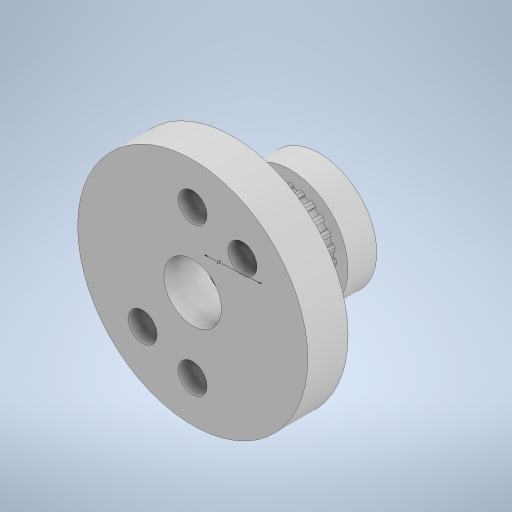
# Autodesk Inventor part: dondurgec
Saved by Autodesk Inventor 2023.2 (Build 272271000, 271)
## iProperties
Created: 2023-03-22
Part Number: dondurgec
Material: Generic
Document SubType Name: Modeling
Designer: sarp1
Density: 1 g/cm^3
Appearance: Default
Author: sarp1
Autodesk Inventor part; units mm, degrees
ref_plane "YZ Plane" through (0, 0, 0) normal (1, 0, 0) x (0, 1, 0)
ref_plane "XZ Plane" through (0, 0, 0) normal (0, 1, 0) x (-1, 0, 0)
ref_plane "XY Plane" through (0, 0, 0) normal (0, 0, 1) x (1, 0, 0)
sketch "Sketch1" plane through (0, 0, 0) normal (0, 0, 1) x (1, 0, 0)
  circle A0 centre (0, 0) radius 20
  circle A1 centre (0, 0) radius 5
  dimension "d0" = 40
  dimension "d1" = 10
  constraints: 2 centre point, 2 coincident
  measures "d0" diameter of A0
  measures "d1" diameter of A1
extrude "Extrusion1" add sketch "Sketch1" along normal blind 5 and the other way blind 2
sketch "Sketch2" plane through (0, 0, 5) normal (0, 0, 1) x (1, 0, 0)
  circle A0 centre (0, 0) radius 5 projected
  line L0 (0, 0) -> (0, 12.85)
  circle A1 centre (0, 12.85) radius 2.5
  line L1 (0, 0) -> (8.6813, 9.474)
  circle A2 centre (8.6813, 9.474) radius 2.5
  circle A3 centre (0, 0) radius 20 projected
  line L2 (0, 0) -> (-20, 0)
  line L3 (0, 0) -> (20, 0) construction
  line L4 (0, 0) -> (-8.6813, -9.474)
  line L5 (0, 0) -> (12.85, 0) construction
  circle A4 centre (-8.6813, -9.474) radius 2.5
  line L6 (0, 0) -> (0, -12.85)
  circle A5 centre (0, -12.85) radius 2.5
  dimension "d4" = 12.85
  dimension "d5" = 5
  dimension "d6" = 12.85
  dimension "d8" = 5
  dimension "d15" = 90
  dimension "d17" = 47.5
  dimension "d18" = 42.5
  dimension "d20" = 12.85
  dimension "d21" = 132.5
  dimension "d22" = 5
  dimension "d23" = 12.85
  dimension "d24" = 5
  dimension "d25" = 42.5
  constraints: 14 end point, 4 centre point, 4 coincident, 3 horizontal, 1 equal length, 1 horizontal alignment, 1 perpendicular, 1 vertical, 1 other
  measures "d4" distance of L0.start L0.end
  measures "d5" diameter of A1
  measures "d6" distance of L0.start L1.end
  measures "d8" diameter of A2
  measures "d15" angle of L2 L0
  measures "d17" angle of L2 L1
  measures "d18" angle of L1 L0
  measures "d20" distance of L2.start L4.end
  measures "d21" angle of L4 L5
  measures "d22" diameter of A4
  measures "d23" distance of L2.start L6.end
  measures "d24" diameter of A5
  measures "d25" angle of L6 L4
extrude "Extrusion2" cut sketch "Sketch2" against normal blind 5 contours A1 | A2 | A4 | A5
sketch "Sketch5" plane through (0, 0, -2) normal (0, 0, -1) x (-1, 0, 0)
  circle A0 centre (0, 0) radius 20 projected
  circle A1 centre (0, 0) radius 5 projected
  circle A2 centre (0, 0) radius 20 projected
  circle A3 centre (0, 0) radius 5 projected
  circle A4 centre (0, 0) radius 5 projected
  circle A5 centre (0, 0) radius 7.5
  circle A6 centre (0, 0) radius 5
  dimension "d34" = 15
  dimension "d35" = 10
  constraints: 2 centre point, 2 coincident
  measures "d34" diameter of A5
  measures "d35" diameter of A6
extrude "Extrusion4" add sketch "Sketch5" along normal blind 10 contours A5
sketch "Sketch6" plane through (0, 0, -12) normal (0, 0, -1) x (-1, 0, 0)
  point P0 (0, 0)
sketch "Sketch7" plane through (0, 0, -2) normal (0, 0, -1) x (-1, 0, 0)
  circle A0 centre (0, 0) radius 0.5 projected
  circle A1 centre (0, 0) radius 5
  dimension "d38" = 10
  constraints: 1 centre point, 1 coincident
  measures "d38" diameter of A1
sketch "Sketch8" plane through (0, 0, -12) normal (0, 0, -1) x (-1, 0, 0)
  circle A0 centre (0, 0) radius 7.5 projected
  line L0 (0, 7.5) -> (0, 8)
  line L1 (0, 8) -> (0.483, 7.8706)
  line L2 (0.483, 7.8706) -> (0.483, 7.4844)
  line L3 (0, 8) -> (-0.483, 7.8706)
  line L4 (-0.483, 7.8706) -> (-0.483, 7.4844)
  line L5 (-2.5036, 7.4774) -> (-2.4036, 7.1044)
  line L6 (-2.0706, 7.7274) -> (-2.5036, 7.4774)
  line L7 (-2.0706, 7.7274) -> (-1.5706, 7.7274)
  line L8 (-1.5706, 7.7274) -> (-1.4706, 7.3544)
  line L9 (-4.3536, 6.5746) -> (-4.1605, 6.2402)
  line L10 (-4, 6.9282) -> (-4.3536, 6.5746)
  line L11 (-4, 6.9282) -> (-3.517, 7.0576)
  line L12 (-3.517, 7.0576) -> (-3.324, 6.7232)
  line L13 (-5.9069, 5.2238) -> (-5.6338, 4.9508)
  line L14 (-5.6569, 5.6569) -> (-5.9069, 5.2238)
  line L15 (-5.6569, 5.6569) -> (-5.2238, 5.9069)
  line L16 (-5.2238, 5.9069) -> (-4.9508, 5.6338)
  line L17 (-7.0576, 3.517) -> (-6.7232, 3.324)
  line L18 (-6.9282, 4) -> (-7.0576, 3.517)
  line L19 (-6.9282, 4) -> (-6.5746, 4.3536)
  line L20 (-6.5746, 4.3536) -> (-6.2402, 4.1605)
  line L21 (-7.7274, 1.5706) -> (-7.3544, 1.4706)
  line L22 (-7.7274, 2.0706) -> (-7.7274, 1.5706)
  line L23 (-7.7274, 2.0706) -> (-7.4774, 2.5036)
  line L24 (-7.4774, 2.5036) -> (-7.1044, 2.4036)
  line L25 (-7.8706, -0.483) -> (-7.4844, -0.483)
  line L26 (-8, 0) -> (-7.8706, -0.483)
  line L27 (-8, 0) -> (-7.8706, 0.483)
  line L28 (-7.8706, 0.483) -> (-7.4844, 0.483)
  line L29 (-7.4774, -2.5036) -> (-7.1044, -2.4036)
  line L30 (-7.7274, -2.0706) -> (-7.4774, -2.5036)
  line L31 (-7.7274, -2.0706) -> (-7.7274, -1.5706)
  line L32 (-7.7274, -1.5706) -> (-7.3544, -1.4706)
  line L33 (-6.5746, -4.3536) -> (-6.2402, -4.1605)
  line L34 (-6.9282, -4) -> (-6.5746, -4.3536)
  line L35 (-6.9282, -4) -> (-7.0576, -3.517)
  line L36 (-7.0576, -3.517) -> (-6.7232, -3.324)
  line L37 (-5.2238, -5.9069) -> (-4.9508, -5.6338)
  line L38 (-5.6569, -5.6569) -> (-5.2238, -5.9069)
  line L39 (-5.6569, -5.6569) -> (-5.9069, -5.2238)
  line L40 (-5.9069, -5.2238) -> (-5.6338, -4.9508)
  line L41 (-3.517, -7.0576) -> (-3.324, -6.7232)
  line L42 (-4, -6.9282) -> (-3.517, -7.0576)
  line L43 (-4, -6.9282) -> (-4.3536, -6.5746)
  line L44 (-4.3536, -6.5746) -> (-4.1605, -6.2402)
  line L45 (-1.5706, -7.7274) -> (-1.4706, -7.3544)
  line L46 (-2.0706, -7.7274) -> (-1.5706, -7.7274)
  line L47 (-2.0706, -7.7274) -> (-2.5036, -7.4774)
  line L48 (-2.5036, -7.4774) -> (-2.4036, -7.1044)
  line L49 (0.483, -7.8706) -> (0.483, -7.4844)
  line L50 (0, -8) -> (0.483, -7.8706)
  line L51 (0, -8) -> (-0.483, -7.8706)
  line L52 (-0.483, -7.8706) -> (-0.483, -7.4844)
  line L53 (2.5036, -7.4774) -> (2.4036, -7.1044)
  line L54 (2.0706, -7.7274) -> (2.5036, -7.4774)
  line L55 (2.0706, -7.7274) -> (1.5706, -7.7274)
  line L56 (1.5706, -7.7274) -> (1.4706, -7.3544)
  line L57 (4.3536, -6.5746) -> (4.1605, -6.2402)
  line L58 (4, -6.9282) -> (4.3536, -6.5746)
  line L59 (4, -6.9282) -> (3.517, -7.0576)
  line L60 (3.517, -7.0576) -> (3.324, -6.7232)
  line L61 (5.9069, -5.2238) -> (5.6338, -4.9508)
  line L62 (5.6569, -5.6569) -> (5.9069, -5.2238)
  line L63 (5.6569, -5.6569) -> (5.2238, -5.9069)
  line L64 (5.2238, -5.9069) -> (4.9508, -5.6338)
  line L65 (7.0576, -3.517) -> (6.7232, -3.324)
  line L66 (6.9282, -4) -> (7.0576, -3.517)
  line L67 (6.9282, -4) -> (6.5746, -4.3536)
  line L68 (6.5746, -4.3536) -> (6.2402, -4.1605)
  line L69 (7.7274, -1.5706) -> (7.3544, -1.4706)
  line L70 (7.7274, -2.0706) -> (7.7274, -1.5706)
  line L71 (7.7274, -2.0706) -> (7.4774, -2.5036)
  line L72 (7.4774, -2.5036) -> (7.1044, -2.4036)
  line L73 (7.8706, 0.483) -> (7.4844, 0.483)
  line L74 (8, 0) -> (7.8706, 0.483)
  line L75 (8, 0) -> (7.8706, -0.483)
  line L76 (7.8706, -0.483) -> (7.4844, -0.483)
  line L77 (7.4774, 2.5036) -> (7.1044, 2.4036)
  line L78 (7.7274, 2.0706) -> (7.4774, 2.5036)
  line L79 (7.7274, 2.0706) -> (7.7274, 1.5706)
  line L80 (7.7274, 1.5706) -> (7.3544, 1.4706)
  line L81 (6.5746, 4.3536) -> (6.2402, 4.1605)
  line L82 (6.9282, 4) -> (6.5746, 4.3536)
  line L83 (6.9282, 4) -> (7.0576, 3.517)
  line L84 (7.0576, 3.517) -> (6.7232, 3.324)
  line L85 (5.2238, 5.9069) -> (4.9508, 5.6338)
  line L86 (5.6569, 5.6569) -> (5.2238, 5.9069)
  line L87 (5.6569, 5.6569) -> (5.9069, 5.2238)
  line L88 (5.9069, 5.2238) -> (5.6338, 4.9508)
  line L89 (3.517, 7.0576) -> (3.324, 6.7232)
  line L90 (4, 6.9282) -> (3.517, 7.0576)
  line L91 (4, 6.9282) -> (4.3536, 6.5746)
  line L92 (4.3536, 6.5746) -> (4.1605, 6.2402)
  line L93 (1.5706, 7.7274) -> (1.4706, 7.3544)
  line L94 (2.0706, 7.7274) -> (1.5706, 7.7274)
  line L95 (2.0706, 7.7274) -> (2.5036, 7.4774)
  line L96 (2.5036, 7.4774) -> (2.4036, 7.1044)
  dimension "d39" = 0.5
  dimension "d40" = 0.5
  dimension "d41" = 75
  dimension "d42" = 0.5
  dimension "d45" = 360
  constraints: 194 end point, 2 parallel, 1 coincident, 1 vertical, 221 other
  measures "d39" distance of L0.start L0.end
  measures "d40" distance of L0.end L1.end
  measures "d41" angle of L0 L1
  measures "d42" distance of L0.end L3.end
extrude "Extrusion5" add sketch "Sketch8" against normal blind 10 contours A0 L73 L74 L75 L76 | A0 L77 L78 L79 L80 | L69 L70 L71 L72 A0 | A0 L81 L82 L83 L84 | L65 L66 L67 L68 A0 | A0 L85 L86 L87 L88 | L61 L62 L63 L64 A0 | A0 L89 L90 L91 L92 | L57 L58 L59 L60 A0 | A0 L93 L94 L95 L96 | L53 L54 L55 L56 A0 | A0 L0 L1 L2 | L49 L50 L51 L52 A0 | A0 L4 L3 L0 | L45 L46 L47 L48 A0 | A0 L5 L6 L7 L8 | L41 L42 L43 L44 A0 | A0 L9 L10 L11 L12 | L37 L38 L39 L40 A0 | A0 L13 L14 L15 L16 | L33 L34 L35 L36 A0 | A0 L17 L18 L19 L20 | L29 L30 L31 L32 A0 | A0 L21 L22 L23 L24 | L25 L26 L27 L28 A0
sketch "Sketch9" plane through (0, 0, -12) normal (0, 0, -1) x (-1, 0, 0)
  circle A0 centre (0, 0) radius 10
  circle A1 centre (0, 0) radius 5 projected
  circle A2 centre (0, 0) radius 5
  dimension "d49" = 20
  constraints: 2 centre point, 2 coincident
  measures "d49" diameter of A0
extrude "Extrusion6" add sketch "Sketch9" along normal blind 5
sketch "Sketch10" plane through (0, 0, -2) normal (0, 0, -1) x (-1, 0, 0)
  point P0 (0, 0)
body "Solid1"
